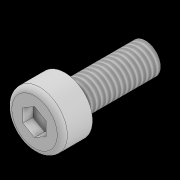
# Autodesk Inventor part: MachineScrew_Template
Saved by Autodesk Inventor 2022.2 (Build 262287010, 287A)
## iProperties
Created: 2022-05-24
Part Number: MachineScrew_Template
Material: Generic
Document SubType Name: Modeling
Designer: Árni Þór Þorgeirsson
Density: 1 g/cm^3
Appearance: Default
Author: Árni Þór Þorgeirsson
Autodesk Inventor part; units mm, degrees
ref_plane "YZ Plane" through (0, 0, 0) normal (1, 0, 0) x (0, 1, 0)
ref_plane "XZ Plane" through (0, 0, 0) normal (0, 1, 0) x (-1, 0, 0)
ref_plane "XY Plane" through (0, 0, 0) normal (0, 0, 1) x (1, 0, 0)
sketch "Sketch3" plane through (0, 0, 0) normal (0, 0, 1) x (1, 0, 0)
  circle A0 centre (0, 0) radius 2.75
  circle A1 centre (0, 0) radius 1.5
  line L0 (1.15, -0.664) -> (0, -1.3279)
  line L1 (0, -1.3279) -> (-1.15, -0.664)
  line L2 (-1.15, -0.664) -> (-1.15, 0.664)
  line L3 (-1.15, 0.664) -> (0, 1.3279)
  line L4 (0, 1.3279) -> (1.15, 0.664)
  line L5 (1.15, 0.664) -> (1.15, -0.664)
  point P0 (1.15, 0)
  dimension "d8" = 1.5
  dimension "d9" = 2.75
  dimension "d10" = 2.3
  constraints: 12 end point, 3 coincident, 2 centre point, 1 midpoint, 13 other
  measures "d8" radius of A1
  measures "d9" radius of A0
  measures "d10" distance from line of point (1.15, 0) L2
extrude "Extrusion1" add sketch "Sketch3" along normal blind 3 contours A0 | A1 | L0 L1 L2 L3 L4 L5
extrude "Extrusion2" add sketch "Sketch3" against normal blind 8 contours A1 | L0 L1 L2 L3 L4 L5
extrude "Extrusion3" cut sketch "Sketch3" against normal blind 1 from surface at 3 contours L0 L1 L2 L3 L4 L5
fillet "Fillet1" radius 0.5 1 edges at (-2.75, 0, 3)
thread "Thread2" size "M3x0.5" class "6g" standard "ISO Metric profile" full length
equation "\"d8\" = 0.5 * Machine_Screw_M"
equation "\"d9\" = Machine_Screw_Head_Radius"
equation "\"d10\" = Machine_Screw_Hex"
equation "\"d11\" = Machine_Screw_Head_Dept"
equation "\"d13\" = Machine_Screw_Length"
equation "\"Machine_Screw_Head_Radius\" = 2.75"
equation "\"Machine_Screw_Head_Dept\" = 3"
equation "\"Machine_Screw_Hex\" = 2.3"
equation "\"Machine_Screw_Length\" = 8"
equation "\"Machine_Screw_M\" = 3"
body "Solid2"
